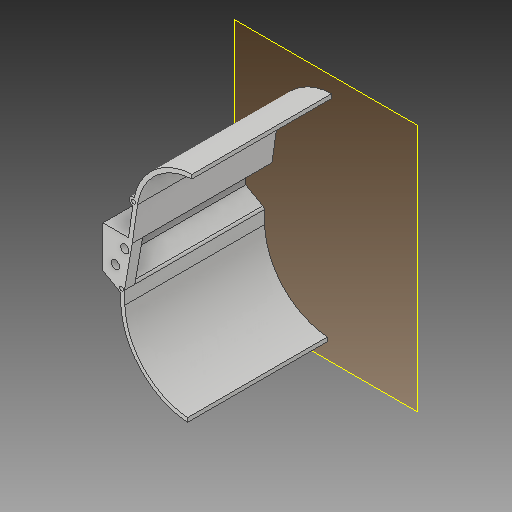
# Autodesk Inventor part: case top half
Saved by Autodesk Inventor 2017 (Build 210142000, 142)
## iProperties
Created: 2018-04-17
Part Number: case top half
Material: Generic
Document SubType Name: Modeling
Designer: RKL
Density: 1 g/cm^3
Appearance: Default
Author: RKL
Autodesk Inventor part; units mm, degrees
ref_plane "YZ Plane" through (0, 0, 0) normal (1, 0, 0) x (0, 1, 0)
ref_plane "XZ Plane" through (0, 0, 0) normal (0, 1, 0) x (-1, 0, 0)
ref_plane "XY Plane" through (0, 0, 0) normal (0, 0, 1) x (1, 0, 0)
ref_plane "Work Plane1" through (0, 0, 0) normal (0, 0, 1) x (1, 0, 0)
sketch "Sketch1" plane through (0, 0, 0) normal (0, 0, 1) x (1, 0, 0)
  circle A0 centre (-55.8916, -14.7421) radius 1.397 projected
  circle A1 centre (-83.8916, 18.2579) radius 1.397 construction
  circle A2 centre (-83.8916, -14.7421) radius 1.397 construction
  circle A3 centre (-55.8916, 18.2579) radius 1.397 projected
  circle A4 centre (2.1895, 105.4705) radius 1.905 projected
  circle A5 centre (-2.169, -104.4843) radius 1.905 projected
  circle A6 centre (60.6164, 51.7463) radius 1.905 projected
  circle A7 centre (-58.4167, 54.2173) radius 1.905 projected
  arc A8 (6.1836, 105.2542) -> (-1.8102, 105.4201) centre (2.1895, 105.4705) ccw projected
  arc A9 (-1.8102, 105.4201) -> (-57.7029, 58.1531) centre (0.9442, 45.4834) ccw projected
  arc A10 (-57.7029, 58.1531) -> (-58.999, 50.2599) centre (-58.4167, 54.2173) ccw projected
  line L0 (-58.999, 50.2599) -> (-63.1925, 21.7579) projected
  line L1 (-87.8916, 21.7579) -> (-63.1925, 21.7579) projected
  line L2 (-87.8916, -18.2421) -> (-87.8916, 21.7579) projected
  line L3 (-87.8916, -18.2421) -> (-73.1277, -26.766) projected
  arc A11 (-73.1277, -26.766) -> (-70.4395, -28.2823) centre (-69.9706, -24.3098) ccw projected
  arc A12 (-70.4395, -28.2823) -> (-6.1641, -104.2871) centre (-0.7162, -34.4994) ccw projected
  arc A13 (-6.1641, -104.2871) -> (1.8309, -104.453) centre (-2.169, -104.4843) ccw projected
  arc A14 (1.8309, -104.453) -> (69.2051, -31.1811) centre (-0.7162, -34.4994) ccw projected
  arc A15 (69.2051, -31.1811) -> (68.4839, -23.2145) centre (68.9014, -27.1927) ccw projected
  line L4 (68.4839, -23.2145) -> (61.034, 47.7681) projected
  arc A16 (61.034, 47.7681) -> (60.0665, 55.7083) centre (60.6164, 51.7463) ccw projected
  arc A17 (60.0665, 55.7083) -> (6.1836, 105.2542) centre (0.9442, 45.4834) ccw projected
  circle A18 centre (-69.9706, -24.3098) radius 1.905 projected
  circle A19 centre (68.9014, -27.1927) radius 1.905 projected
  circle A20 centre (0.9442, 45.4834) radius 17.5 projected
  circle A21 centre (-0.7162, -34.4994) radius 17.5 projected
  circle A22 centre (-66.7556, 10.6536) radius 4 projected
  circle A23 centre (-75.8916, -7.1378) radius 4 projected
  circle A24 centre (68.9014, -27.1927) radius 1.905 construction
  circle A25 centre (60.6164, 51.7463) radius 1.905 construction
  circle A26 centre (-2.169, -104.4843) radius 1.905 construction
  circle A27 centre (2.1895, 105.4705) radius 1.905 construction
  arc A28 (6.1836, 105.2542) -> (-1.8102, 105.4201) centre (2.1895, 105.4705) ccw construction
  arc A29 (60.0665, 55.7083) -> (6.1836, 105.2542) centre (0.9442, 45.4834) ccw construction
  arc A30 (61.034, 47.7681) -> (60.0665, 55.7083) centre (60.6164, 51.7463) ccw construction
  line L5 (61.034, 47.7681) -> (68.4839, -23.2145) construction
  arc A31 (69.2051, -31.1811) -> (68.4839, -23.2145) centre (68.9014, -27.1927) ccw construction
  arc A32 (1.8309, -104.453) -> (69.2051, -31.1811) centre (-0.7162, -34.4994) ccw construction
  arc A33 (-6.1641, -104.2871) -> (1.8309, -104.453) centre (-2.169, -104.4843) ccw construction
  line L6 (-6.1641, -104.2871) -> (-6.0811, -100.2871) construction
  arc A34 (-6.0811, -100.2871) -> (64.9295, -27.6117) centre (-0.7162, -34.4994) ccw construction
  line L7 (64.9295, -27.6117) -> (56.6471, 51.3278) construction
  arc A35 (56.6471, 51.3278) -> (-1.8933, 101.4201) centre (0.9442, 45.4834) ccw construction
  line L8 (-1.8933, 101.4201) -> (-1.8102, 105.4201) construction
  line L9 (-6.1641, -104.2871) -> (-6.0811, -100.2871)
  line L10 (-1.8933, 101.4201) -> (-1.8102, 105.4201)
  arc A36 (-1.8933, 101.4201) -> (-54.4679, 53.6363) centre (0.9442, 45.4834) ccw
  line L11 (-54.4679, 53.6363) -> (-59.5996, 18.7579)
  line L12 (-59.5996, 18.7579) -> (-84.8916, 18.7579)
  line L13 (-84.8916, 18.7579) -> (-84.8916, -12.3408)
  arc A37 (-66.6915, -36.5144) -> (-6.0811, -100.2871) centre (-0.7162, -34.4994) ccw
  arc A38 (-67.0669, -24.2212) -> (-68.5181, -21.794) centre (-69.9706, -24.3098) ccw
  line L14 (-66.6915, -36.5144) -> (-67.0669, -24.2212)
  line L15 (-84.8916, -12.3408) -> (-68.5181, -21.794)
  point P0 (0, 0)
  dimension "d0" = 1
  dimension "d1" = 3
  dimension "d2" = 3
  constraints: 14 end point, 6 point on circle, 4 parallel, 4 tangent, 3 centre point, 3 coincident, 2 collinear, 1 horizontal
  measures "d0" radial gap between concentric circles of A18 A38
  measures "d1" distance between parallel lines of L2 L13
  measures "d2" distance between parallel lines of L1 L12
extrude "Extrusion1" add sketch "Sketch1" along normal blind 125 contours L10 A36 L11 L12 L13 L15 A38 L14 A37 L9 A12 A11 L3 L2 L1 L0 A10 A9
sketch "Sketch2" plane through (0, 0, 125) normal (0, 0, 1) x (1, 0, 0)
  circle A0 centre (-69.9706, -24.3098) radius 1.905 projected
  circle A1 centre (-58.4167, 54.2173) radius 1.905 projected
  arc A2 (-1.8102, 105.4201) -> (-57.7029, 58.1531) centre (0.9442, 45.4834) ccw projected
  arc A3 (-57.7029, 58.1531) -> (-58.999, 50.2599) centre (-58.4167, 54.2173) ccw projected
  line L0 (-58.999, 50.2599) -> (-63.1925, 21.7579) projected
  line L1 (-63.1925, 21.7579) -> (-87.8916, 21.7579) projected
  line L2 (-87.8916, 21.7579) -> (-87.8916, -18.2421) projected
  line L3 (-87.8916, -18.2421) -> (-73.1277, -26.766) projected
  arc A4 (-73.1277, -26.766) -> (-70.4395, -28.2823) centre (-69.9706, -24.3098) ccw projected
  arc A5 (-70.4395, -28.2823) -> (-6.1641, -104.2871) centre (-0.7162, -34.4994) ccw projected
  line L4 (-6.1641, -104.2871) -> (-6.0811, -100.2871) projected
  arc A6 (-66.6915, -36.5144) -> (-6.0811, -100.2871) centre (-0.7162, -34.4994) ccw projected
  line L5 (-66.6915, -36.5144) -> (-67.0669, -24.2212) projected
  arc A7 (-67.0669, -24.2212) -> (-68.5181, -21.794) centre (-69.9706, -24.3098) ccw projected
  line L6 (-68.5181, -21.794) -> (-84.8916, -12.3408) projected
  line L7 (-84.8916, -12.3408) -> (-84.8916, 18.7579) projected
  line L8 (-84.8916, 18.7579) -> (-59.5996, 18.7579) projected
  line L9 (-59.5996, 18.7579) -> (-54.4679, 53.6363) projected
  arc A8 (-1.8933, 101.4201) -> (-54.4679, 53.6363) centre (0.9442, 45.4834) ccw projected
  line L10 (-1.8933, 101.4201) -> (-1.8102, 105.4201) projected
  circle A9 centre (-66.7556, 10.6536) radius 4 projected
  circle A10 centre (-75.8916, -7.1378) radius 4 projected
  line L11 (-66.6915, -36.5144) -> (-67.0669, -24.2212) projected
  line L12 (-59.5996, 18.7579) -> (-67.0669, -24.2212)
  point P0 (0, 0)
  constraints: 2 end point
ref_plane "Work Plane2" through (-78.4932, -111.5319, 135) normal (0, 0, -1) x (0, 1, 0)
extrude "Extrusion2" add sketch "Sketch2" along normal up to surface (10 mm away)
body "Solid1"
